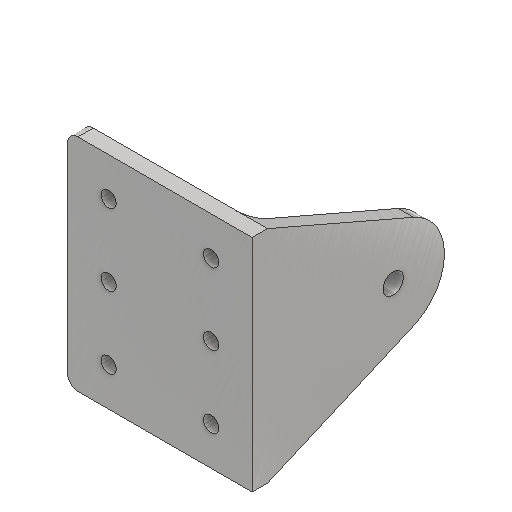
# Autodesk Inventor part: CNCM_ALU_X_Axis_Idler_Mounting_Bracket
Saved by Autodesk Inventor 2026.1 (Build 301233000, 233)
## iProperties
Created: 2016-03-27
Part Number: CNCM_ALU_X_Axis_Idler_Mounting_Bracket
Material: Ogólny
Document SubType Name: Modeling
Designer: Andrzej
Density: 1 g/cm^3
Appearance: Obrobione - aluminium
Mass: 7.42996 g
Surface Area: 56.0163 cm^2
Volume: 7.42996 cm^3
Author: Andrzej
Autodesk Inventor part; units mm, degrees
ref_plane "YZ Plane" through (0, 0, 0) normal (1, 0, 0) x (0, 1, 0)
ref_plane "XZ Plane" through (0, 0, 0) normal (0, 1, 0) x (-1, 0, 0)
ref_plane "XY Plane" through (0, 0, 0) normal (0, 0, 1) x (1, 0, 0)
sketch "Szkic1" plane through (0, 0, 0) normal (0, 0, 1) x (1, 0, 0)
  line L0 (-15.1556, -3.6171) -> (-15.1556, -6.6171)
  line L1 (-15.1556, -6.6171) -> (20.8444, -6.6171)
  line L2 (20.8444, -6.6171) -> (20.8444, 40.3829)
  line L3 (20.8444, 40.3829) -> (17.8444, 40.3829)
  line L4 (17.8444, 40.3829) -> (17.8444, -3.6171)
  line L5 (17.8444, -3.6171) -> (-15.1556, -3.6171)
  point P0 (0, 0)
  dimension "d0" = 3
  dimension "d1" = 36
  dimension "d2" = 47
  dimension "d3" = 3
  constraints: 12 end point, 5 perpendicular, 1 vertical
  measures "d0" distance of L0.start L0.end
  measures "d1" distance of L0.end L1.end
  measures "d2" distance of L1.end L2.end
  measures "d3" distance of L2.end L3.end
extrude "Wyciągnięcie proste1" add sketch "Szkic1" along normal blind 43
fillet "Zaokrąglenie1" radius 3 1 edges at (17.8444, -3.6171, 21.5)
fillet "Zaokrąglenie2" radius 2 2 edges at (-15.1556, -5.1171, 0) (-15.1556, -5.1171, 43)
sketch "Szkic3" plane through (20.8444, -6.6171, 0) normal (0, -1, 0) x (1, 0, 0)
  arc A0 (-34, 43) -> (-36, 41) centre (-34, 41) ccw projected
  line L0 (-36, 2) -> (-36, 41) projected
  arc A1 (-36, 2) -> (-34, 0) centre (-34, 2) ccw projected
  line L1 (-34, 0) -> (0, 0) projected
  line L2 (0, 0) -> (0, 43) projected
  line L3 (-34, 43) -> (0, 43) projected
  point P0 (-20.8444, 0)
  point P1 (-28, 35.5)
  point P2 (-8, 35.5)
  point P3 (-28, 7.5)
  point P4 (-8, 7.5)
  dimension "d40" = 20
  dimension "d41" = 20
  dimension "d42" = 36
  dimension "d43" = 8
  dimension "d44" = 8
  dimension "d45" = 7.5
  dimension "d46" = 7.5
  dimension "d47" = 7.5
  dimension "d48" = 7.5
  measures "d40" distance of point (-8, 35.5) point (-28, 35.5)
  measures "d41" distance of point (-8, 7.5) point (-28, 7.5)
  measures "d42" distance between parallel lines of L2 L0
  measures "d43" distance from line of L0 point (-28, 35.5)
  measures "d44" distance from line of L0 point (-28, 7.5)
  measures "d45" distance from line of L3 point (-28, 35.5)
  measures "d46" distance from line of L3 point (-8, 35.5)
  measures "d47" distance from line of L1 point (-28, 7.5)
  measures "d48" distance from line of L1 point (-8, 7.5)
hole "Otwór3" at (-7.1556, -6.6171, 35.5) at (12.8444, -6.6171, 35.5) at (-7.1556, -6.6171, 7.5) at (12.8444, -6.6171, 7.5) direction (0, 1, 0) diameter 3 end through all
sketch "Szkic4" plane through (20.8444, -6.6171, 0) normal (1, 0, 0) x (0, 0, -1)
  line L0 (0, 0) -> (0, 47) projected
  line L1 (0, 47) -> (-43, 47) projected
  line L2 (-43, 0) -> (-43, 47) projected
  line L3 (0, 0) -> (-43, 0) projected
  line L4 (0, 3) -> (-43, 3) projected
  circle A0 centre (-21.5, 27.5) radius 10
  line L5 (-43, 3) -> (-30.6773, 31.472)
  line L6 (0, 3) -> (-12.3227, 31.472)
  point P0 (0, 6.6171)
  dimension "d57" = 43
  dimension "d58" = 21.5
  dimension "d59" = 27.5
  dimension "d60" = 20
  constraints: 4 end point, 2 point on circle, 2 tangent, 1 centre point, 1 coincident
  measures "d57" distance between parallel lines of L0 L2
  measures "d58" distance from line of L2 point (-21.5, 27.5)
  measures "d59" distance from line of L3 point (-21.5, 27.5)
  measures "d60" diameter of A0
extrude "Wyciągnięcie proste4" cut sketch "Szkic4" against normal blind 10 contours L6 A0 L5 L2 L1 L0
hole "Otwór4" at (20.8444, 20.8829, 21.5) direction (-1, 0, 0) diameter 4 end through all
sketch "Szkic5" plane through (-15.1556, -3.6171, 41) normal (0, 1, 0) x (1, 0, 0)
  circle A0 centre (28, 5.5) radius 1.5 projected
  circle A1 centre (28, 33.5) radius 1.5 projected
  circle A2 centre (28, 5.5) radius 3.1
  circle A3 centre (28, 33.5) radius 1.5 projected
  circle A4 centre (28, 33.5) radius 3.1
  point P0 (15.1556, 41)
  dimension "d70" = 6.2
  dimension "d71" = 6.2
  constraints: 2 centre point, 2 coincident
  measures "d70" diameter of A2
  measures "d71" diameter of A4
extrude "Wyciągnięcie proste5" cut sketch "Szkic5" along normal blind 10
sketch "Szkic6" plane through (20.8444, -6.6171, 0) normal (0, -1, 0) x (1, 0, 0)
  circle A0 centre (-28, 7.5) radius 1.5 projected
  circle A1 centre (-28, 35.5) radius 1.5 projected
  circle A2 centre (-8, 35.5) radius 1.5 projected
  circle A3 centre (-8, 7.5) radius 1.5 projected
  arc A4 (-34, 43) -> (-36, 41) centre (-34, 41) ccw projected
  line L0 (-36, 2) -> (-36, 41) projected
  arc A5 (-36, 2) -> (-34, 0) centre (-34, 2) ccw projected
  line L1 (-34, 0) -> (0, 0) projected
  line L2 (0, 0) -> (0, 43) projected
  line L3 (-34, 43) -> (0, 43) projected
  point P0 (-20.8444, 0)
  point P1 (-28, 21.5)
  point P2 (-8, 21.5)
  dimension "d74" = 14
  dimension "d75" = 14
  dimension "d76" = 14
  dimension "d77" = 14
  measures "d74" distance of A1.centre point (-28, 21.5)
  measures "d75" distance of A0.centre point (-28, 21.5)
  measures "d76" distance of A3.centre point (-8, 21.5)
  measures "d77" distance of A2.centre point (-8, 21.5)
hole "Otwór5" at (-7.1556, -6.6171, 21.5) at (12.8444, -6.6171, 21.5) direction (0, 1, 0) diameter 3 end through all
equation "\"d41\" = d40"
equation "\"d43\" = -0.5 * d40 + 0.5 * d42"
equation "\"d44\" = d43"
equation "\"d46\" = d45"
equation "\"d47\" = d45"
equation "\"d48\" = d47"
equation "\"d58\" = 0.5 * d57"
